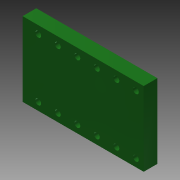
# Autodesk Inventor part: 知能ロボコンギアボックススペーサ
Saved by Autodesk Inventor 2013 (Build 170138000, 138)
## iProperties
Created: 2014-08-21
Part Number: 知能ロボコンギアボックススペーサ
Material: ABS プラスチック
Document SubType Name: Modeling
Designer: horumo136
Density: 1 g/cm^3
Author: horumo136
Autodesk Inventor part; units mm, degrees
ref_plane "YZ Plane" through (0, 0, 0) normal (1, 0, 0) x (0, 1, 0)
ref_plane "XZ Plane" through (0, 0, 0) normal (0, 1, 0) x (-1, 0, 0)
ref_plane "XY Plane" through (0, 0, 0) normal (0, 0, 1) x (1, 0, 0)
sketch "スケッチ1" plane through (0, 0, 0) normal (0, 1, 0) x (-1, 0, 0)
  line L0 (0, 0) -> (-62, 0)
  line L1 (-62, 0) -> (-62, 38)
  line L2 (-62, 38) -> (0, 38)
  line L3 (0, 38) -> (0, 0)
  line L4 (0, 19) -> (-8, 19)
  line L5 (-8, 19) -> (-8, 34)
  line L6 (-8, 34) -> (-18, 34)
  line L7 (-18, 34) -> (-28, 34)
  line L8 (-28, 34) -> (-38, 34)
  line L9 (-38, 34) -> (-48, 34)
  line L10 (-48, 34) -> (-58, 34)
  line L11 (-8, 4) -> (-18, 4)
  line L12 (-18, 4) -> (-28, 4)
  line L13 (-28, 4) -> (-38, 4)
  line L14 (-38, 4) -> (-48, 4)
  line L15 (-48, 4) -> (-58, 4)
  circle A0 centre (-58, 34) radius 1.5
  circle A1 centre (-48, 34) radius 1.5
  circle A2 centre (-38, 34) radius 1.5
  circle A3 centre (-28, 34) radius 1.5
  circle A4 centre (-18, 34) radius 1.5
  circle A5 centre (-8, 34) radius 1.5
  circle A6 centre (-58, 4) radius 1.5
  circle A7 centre (-48, 4) radius 1.5
  circle A8 centre (-38, 4) radius 1.5
  circle A9 centre (-28, 4) radius 1.5
  circle A10 centre (-18, 4) radius 1.5
  circle A11 centre (-8, 4) radius 1.5
  dimension "d0" = 62
  dimension "d1" = 38
  dimension "d2" = 8
  dimension "d3" = 15
  dimension "d4" = 10
  dimension "d5" = 10
  dimension "d6" = 10
  dimension "d7" = 10
  dimension "d8" = 10
  dimension "d9" = 3
  dimension "d10" = 3
  dimension "d11" = 3
  dimension "d12" = 3
  dimension "d13" = 3
  dimension "d14" = 3
  constraints: 32 end point, 18 coincident, 18 symmetric about line, 12 centre point, 7 parallel, 3 perpendicular, 1 horizontal, 1 midpoint, 6 other
  measures "d0" distance of L1.end L2.end
  measures "d1" distance of L0.end L1.end
  measures "d2" distance of L4.start L4.end
  measures "d3" distance of L4.end L5.end
  measures "d4" distance of L5.end L6.end
  measures "d5" distance of L6.end L7.end
  measures "d6" distance of L7.end L8.end
  measures "d7" distance of L8.end L9.end
  measures "d8" distance of L9.end L10.end
  measures "d9" diameter of A0
  measures "d10" diameter of A1
  measures "d11" diameter of A2
  measures "d12" diameter of A3
  measures "d13" diameter of A4
  measures "d14" diameter of A5
extrude "押し出し1" add sketch "スケッチ1" along normal blind 7
